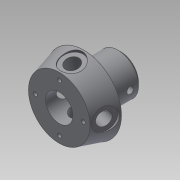
# Autodesk Inventor part: Гайка
Saved by Autodesk Inventor 2014 SP1 (Build 180222100, 222)
## iProperties
Created: 2021-12-02
Part Number: Гайка
Material: Типовые
Document SubType Name: Modeling
Designer: Украинцев
Mass: 42.5324 g
Surface Area: 128.981 cm^2
Volume: 42.5324 cm^3
Density: 1 g/cm^3
Appearance: По умолчанию
Author: Украинцев
Autodesk Inventor part; units mm, degrees
ref_plane "YZ Plane" through (0, 0, 0) normal (1, 0, 0) x (0, 1, 0)
ref_plane "XZ Plane" through (0, 0, 0) normal (0, 1, 0) x (-1, 0, 0)
ref_plane "XY Plane" through (0, 0, 0) normal (0, 0, 1) x (1, 0, 0)
sketch "Эскиз1" plane through (0, 0, 0) normal (0, 0, 1) x (1, 0, 0)
  line L0 (0, 0) -> (22.5, 0)
  line L1 (22.5, 0) -> (27.5, 18)
  line L2 (27.5, 18) -> (15, 25)
  line L3 (15, 25) -> (15, 45)
  line L4 (15, 45) -> (0, 45)
  line L5 (0, 45) -> (0, 0)
  line L6 (25, 9) -> (0, 15.6987)
  line L7 (27.2082, 16.9494) -> (25.2763, 17.467)
  line L8 (25.2763, 17.467) -> (24.4351, 14.3277)
  line L9 (24.4351, 14.3277) -> (0, 20.8751)
  dimension "d0" = 45
  dimension "d1" = 30
  dimension "d2" = 20
  dimension "d3" = 18
  dimension "d4" = 55
  dimension "d5" = 45
  dimension "d14" = 15
  dimension "d15" = 9
  dimension "d16" = 2
  dimension "d17" = 16.5
  dimension "d18" = 10
  constraints: 20 end point, 4 parallel, 3 point on line, 2 perpendicular, 1 horizontal, 1 midpoint
  measures "d0" distance of L4.end L0.start
  measures "d1" diameter of L3 L5
  measures "d2" distance of L2.end L3.end
  measures "d3" vertical distance of L1.end L0.end
  measures "d4" diameter of L1.end L5
  measures "d5" vertical distance of L0.end L5
  measures "d14" angle of L6 L0
  measures "d15" vertical distance of L0.end L6.start
  measures "d16" distance of L7.start L7.end
  measures "d17" diameter of L7 L6
  measures "d18" diameter of L9 L6
revolve "Вращение1" add sketch "Эскиз1" angle 360 about axis through (0, 45, 0) along (0, -1, 0)
sketch "Эскиз2" plane through (0, 0, 0) normal (0, -1, 0) x (1, 0, 0)
  point P0 (0, 0)
  point P1 (0, 0)
  constraints: 1 coincident
hole "Отверстие1" at (0, 0, 0) direction (0, 1, 0) diameter 13.835 end through all counterbore diameter 20 counterbore depth 23 thread size "M16x2" class "6H" standard "ISO Metric profile"
revolve "Вращение2" cut sketch "Эскиз1" angle 360 about axis through (25, 9, 0) along (-0.9659258, 0.258819, 0) contours L5 L9 L8 L7 L1 L6
pattern_circular "Круговой массив1" count 4 over 360 about axis through (0, 89.861, 0) along (0, -1, 0) of "Вращение2"
sketch "Эскиз3" plane through (0, 0, 0) normal (1, 0, 0) x (0, 1, 0)
  circle A0 centre (37, 0) radius 2.5
  line L0 (45, 6.9175) -> (45, -6.9175) projected
  point P0 (0, 0)
  dimension "d23" = 5
  dimension "d24" = 8
  constraints: 1 centre point, 1 horizontal alignment
  measures "d23" diameter of A0
  measures "d24" distance from line of L0 A0.centre
extrude "Выдавливание1" cut sketch "Эскиз3" along normal through all both and the other way through all
sketch "Эскиз4" plane through (0, 0, 0) normal (0, -1, 0) x (1, 0, 0)
  circle A0 centre (17.5, 0) radius 1.5
  circle A1 centre (0, 0) radius 17.5 construction
  dimension "d27" = 35
  dimension "d28" = 3
  constraints: 2 horizontal alignment, 1 centre point, 1 coincident, 2 other
  measures "d28" diameter of A0
extrude "Выдавливание2" cut sketch "Эскиз4" against normal through all
pattern_circular "Круговой массив2" count 4 over 360 about axis through (0, 11.5, 0) along (0, -1, 0) of "Выдавливание2"
chamfer "Фаска1" distance 1.6 angle 45 2 edges at (0, 45, 6.9175) (0, 23, 6.9175)
chamfer "Фаска2" distance 2 angle 45 1 edges at (-15, 45, 0)
